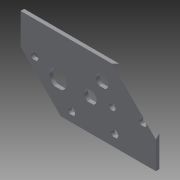
# Autodesk Inventor part: DishFront_BackPlate
Saved by Autodesk Inventor 2014 (Build 180170000, 170)
## iProperties
Created: 2015-01-07
Part Number: DishFront_BackPlate
Material: Generic
Document SubType Name: Modeling
Designer: Owner
Density: 1 g/cm^3
Appearance: Default
Author: Owner
Autodesk Inventor part; units mm, degrees
ref_plane "YZ Plane" through (0, 0, 0) normal (1, 0, 0) x (0, 1, 0)
ref_plane "XZ Plane" through (0, 0, 0) normal (0, 1, 0) x (-1, 0, 0)
ref_plane "XY Plane" through (0, 0, 0) normal (0, 0, 1) x (1, 0, 0)
sketch "Sketch1" plane through (0, 0, 0) normal (0, 0, 1) x (1, 0, 0)
  line L0 (-131.3923, -13.6452) -> (-10.7423, -13.6452)
  line L1 (-10.7423, -13.6452) -> (-10.7423, -77.1452)
  line L2 (-10.7423, -77.1452) -> (-131.3923, -77.1452)
  line L3 (-131.3923, -77.1452) -> (-131.3923, -13.6452)
  point P0 (0, 0)
  dimension "d0" = 120.65
  dimension "d1" = 63.5
  constraints: 8 end point, 2 parallel, 1 horizontal, 1 perpendicular
  measures "d0" distance of L0.start L0.end
  measures "d1" distance of L0.end L1.end
extrude "Extrusion1" add sketch "Sketch1" along normal blind 3.175
sketch "Sketch2" plane through (0, 0, 3.175) normal (0, 0, 1) x (1, 0, 0)
  line L0 (-131.3923, -77.1452) -> (-10.7423, -77.1452) projected
  line L1 (-10.7423, -13.6452) -> (-131.3923, -13.6452) projected
  circle A0 centre (-97.9865, -49.6104) radius 10.3124 construction
  arc A1 (-94.744, -56.6462) -> (-101.2289, -56.6462) centre (-97.9865, -49.6104) ccw
  circle A2 centre (-69.0552, -48.9507) radius 9.0932 construction
  arc A3 (-66.3161, -53.6751) -> (-71.7943, -53.6751) centre (-69.0552, -48.9507) ccw
  circle A4 centre (-49.6427, -46.7902) radius 5.2451 construction
  circle A5 centre (-49.6427, -46.7902) radius 2.9464
  line L2 (-101.2289, -56.6462) -> (-94.744, -56.6462)
  line L3 (-71.7943, -53.6751) -> (-66.3161, -53.6751)
  circle A6 centre (-58.5828, -31.608) radius 9.0932 construction
  arc A7 (-55.8437, -36.3324) -> (-61.3218, -36.3324) centre (-58.5828, -31.608) ccw
  line L4 (-61.3218, -36.3324) -> (-55.8437, -36.3324)
  arc A8 (-117.1413, -45.2795) -> (-120.6054, -45.2795) centre (-118.8734, -42.5295) ccw
  line L5 (-117.1413, -45.2795) -> (-120.6054, -45.2795)
  circle A9 centre (-118.8734, -42.5295) radius 5.5 construction
  arc A10 (-84.1844, -71.2418) -> (-87.6485, -71.2418) centre (-85.9164, -68.4918) ccw
  line L6 (-84.1844, -71.2418) -> (-87.6485, -71.2418)
  circle A11 centre (-85.9164, -68.4918) radius 5.5 construction
  arc A12 (-45.8101, -69.4532) -> (-49.2742, -69.4532) centre (-47.5422, -66.7032) ccw
  line L7 (-45.8101, -69.4532) -> (-49.2742, -69.4532)
  circle A13 centre (-47.5422, -66.7032) radius 5.5 construction
  arc A14 (-20.5575, -48.0295) -> (-24.0216, -48.0295) centre (-22.2896, -45.2795) ccw
  line L8 (-20.5575, -48.0295) -> (-24.0216, -48.0295)
  circle A15 centre (-22.2896, -45.2795) radius 5.5 construction
  point P0 (0, 0)
  dimension "d18" = 20.6248
  dimension "d19" = 15.494
  dimension "d20" = 18.1864
  dimension "d21" = 10.922
  dimension "d22" = 10.4902
  dimension "d23" = 5.8928
  dimension "d24" = 7.0358
  dimension "d25" = 4.7244
  dimension "d26" = 18.1864
  dimension "d27" = 10.922
  dimension "d28" = 4.7244
  dimension "d31" = 27.5348
  dimension "d32" = 28.1945
  dimension "d34" = 30.3551
  dimension "d36" = 6.5
  dimension "d37" = 2.75
  dimension "d38" = 11
  dimension "d39" = 6.5
  dimension "d40" = 2.75
  dimension "d41" = 11
  dimension "d42" = 6.5
  dimension "d43" = 2.75
  dimension "d44" = 11
  dimension "d45" = 6.5
  dimension "d46" = 2.75
  dimension "d47" = 11
  constraints: 16 centre point, 14 end point, 14 point on circle, 8 coincident, 7 parallel
  measures "d18" diameter of A0
  measures "d19" diameter of A1
  measures "d20" diameter of A2
  measures "d21" diameter of A3
  measures "d22" diameter of A4
  measures "d23" diameter of A5
  measures "d24" distance from line of L2 A0.centre
  measures "d25" distance from line of L3 A2.centre
  measures "d26" diameter of A6
  measures "d27" diameter of A7
  measures "d28" distance from line of L4 A6.centre
  measures "d31" distance from line of L0 A0.centre
  measures "d32" distance from line of L0 A2.centre
  measures "d34" distance from line of L0 A4.centre
  measures "d36" diameter of A8
  measures "d37" distance from line of L5 A8.centre
  measures "d38" diameter of A9
  measures "d39" diameter of A10
  measures "d40" distance from line of L6 A10.centre
  measures "d41" diameter of A11
  measures "d42" diameter of A12
  measures "d43" distance from line of L7 A12.centre
  measures "d44" diameter of A13
  measures "d45" diameter of A14
  measures "d46" distance from line of L8 A14.centre
  measures "d47" diameter of A15
extrude "Extrusion2" cut sketch "Sketch2" against normal blind 6.35
body "Solid1"
